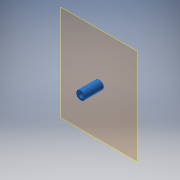
# Autodesk Inventor part: spacer
Saved by Autodesk Inventor 2016 (Build 200138000, 138)
## iProperties
Created: 2016-09-29
Part Number: spacer
Material: Generic
Document SubType Name: Modeling
Designer: benja
Density: 1 g/cm^3
Appearance: Cyan
Author: benja
Autodesk Inventor part; units mm, degrees
ref_plane "YZ Plane" through (0, 0, 0) normal (1, 0, 0) x (0, 1, 0)
ref_plane "XZ Plane" through (0, 0, 0) normal (0, 1, 0) x (-1, 0, 0)
ref_plane "XY Plane" through (0, 0, 0) normal (0, 0, 1) x (1, 0, 0)
ref_plane "Work Plane1" through (9.6073, -5.465, 0) normal (0, 0, 1) x (1, 0, 0)
sketch "Sketch1" plane through (9.6073, -5.465, 0) normal (0, 0, 1) x (1, 0, 0)
  circle A0 centre (-9.6073, 5.465) radius 1.75
  circle A1 centre (-9.6073, 5.465) radius 3.75
  dimension "d0" = 3.5
  dimension "d1" = 2
  constraints: 2 centre point, 2 coincident
  measures "d0" diameter of A0
  measures "d1" radial gap between concentric circles of A0 A1
extrude "Extrusion1" add sketch "Sketch1" along normal blind 14
body "Solid1"
